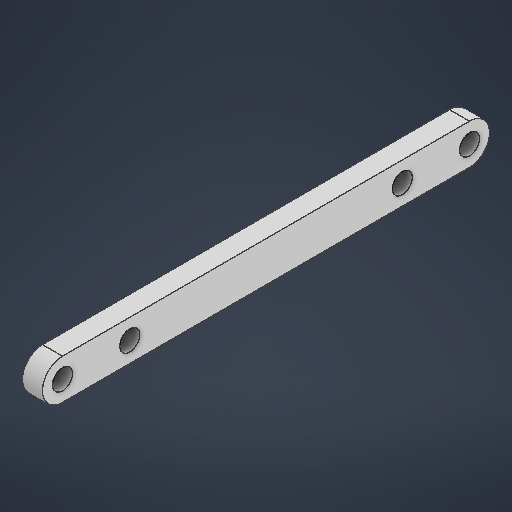
# Autodesk Inventor part: wago_support_support
Saved by Autodesk Inventor 2026.1 (Build 301233000, 233)
## iProperties
Created: 2026-05-05
Part Number: wago_support_support
Material: Generic
Document SubType Name: Modeling
Designer: emanuel
Density: 1 g/cm^3
Appearance: Default
Author: emanuel
Autodesk Inventor part; units mm, degrees
ref_plane "YZ Plane" through (0, 0, 0) normal (1, 0, 0) x (0, 1, 0)
ref_plane "XZ Plane" through (0, 0, 0) normal (0, 1, 0) x (-1, 0, 0)
ref_plane "XY Plane" through (0, 0, 0) normal (0, 0, 1) x (1, 0, 0)
sketch "Sketch1" plane through (0, 0, 0) normal (1, 0, 0) x (0, 1, 0)
  line L0 (0, -30.5) -> (0, 30.5)
  line L1 (0, 20.422) -> (0, -20.422)
  circle A0 centre (0, 20.422) radius 1.5
  circle A1 centre (0, 30.5) radius 1.5
  circle A2 centre (0, -20.422) radius 1.5
  circle A3 centre (0, -30.5) radius 1.5
  line L2 (0, 30.5) -> (0, -30.5) construction
  line L3 (-3, 30.5) -> (-3, -30.5)
  line L4 (3, -30.5) -> (3, 30.5)
  arc A4 (3, 30.5) -> (-3, 30.5) centre (0, 30.5) ccw
  arc A5 (-3, -30.5) -> (3, -30.5) centre (0, -30.5) ccw
  point P0 (0, 0)
  point P1 (0, 0)
  dimension "d0" = 61
  dimension "d1" = 40.844
  dimension "d2" = 3
  dimension "d3" = 3
  dimension "d4" = 3
  dimension "d5" = 3
  dimension "d6" = 6
  constraints: 12 end point, 6 centre point, 4 coincident, 4 point on circle, 4 tangent, 3 midpoint, 2 vertical, 1 parallel, 1 point on line
  measures "d0" distance of L0.start L0.end
  measures "d1" distance of L1.start L1.end
  measures "d2" diameter of A0
  measures "d3" diameter of A1
  measures "d4" diameter of A2
  measures "d5" diameter of A3
  measures "d6" diameter of A5
extrude "Extrusion1" add sketch "Sketch1" along normal blind 3
body "Solid1"
